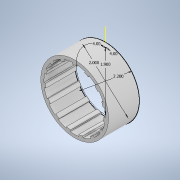
# Autodesk Inventor part: Wheel With Ridges
Saved by Autodesk Inventor 2020 (Build 240168000, 168)
## iProperties
Created: 2020-01-30
Part Number: Wheel With Ridges
Material: Generic
Document SubType Name: Modeling
Designer: cks4a449
Density: 1 g/cm^3
Appearance: Default
Author: cks4a449
Autodesk Inventor part; units mm, degrees
ref_plane "YZ Plane" through (0, 0, 0) normal (1, 0, 0) x (0, 1, 0)
ref_plane "XZ Plane" through (0, 0, 0) normal (0, 1, 0) x (-1, 0, 0)
ref_plane "XY Plane" through (0, 0, 0) normal (0, 0, 1) x (1, 0, 0)
sketch "Sketch1" plane through (0, 0, 0) normal (0, 0, 1) x (1, 0, 0)
  circle A0 centre (0, 0) radius 25.4
  circle A1 centre (0, 0) radius 27.94
  arc A2 (1.6832, 24.0712) -> (-1.6832, 24.0712) centre (0, 0) ccw
  line L0 (1.6832, 24.0712) -> (1.7718, 25.3381)
  line L1 (-1.6832, 24.0712) -> (-1.7718, 25.3381)
  line L2 (0, 39.116) -> (0, -39.116) projected
  dimension "d0" = 50.8
  dimension "d1" = 55.88
  dimension "d4" = 48.26
  dimension "d5" = 4
  dimension "d6" = 4
  constraints: 4 end point, 4 point on circle, 3 centre point, 3 coincident
  measures "d0" diameter of A0
  measures "d1" diameter of A1
  measures "d4" diameter of A2
  measures "d5" angle of L2 L0
  measures "d6" angle of L2 L1
extrude "Extrusion1" add sketch "Sketch1" along normal blind 25.4 contours A0 L2 A1 | L2 A1 A0
extrude "Extrusion2" add sketch "Sketch1" along normal blind 25.4 contours L0 A2 L2 A0 | L2 A2 L1 A0 picked at (0.3842, 24.9722) picked at (-0.3842, 24.9722)
pattern_circular "Circular Pattern1" count 15 over 360 about axis through (0, 0, -10) along (0, 0, 1) of "Extrusion2"
body "Solid1"
